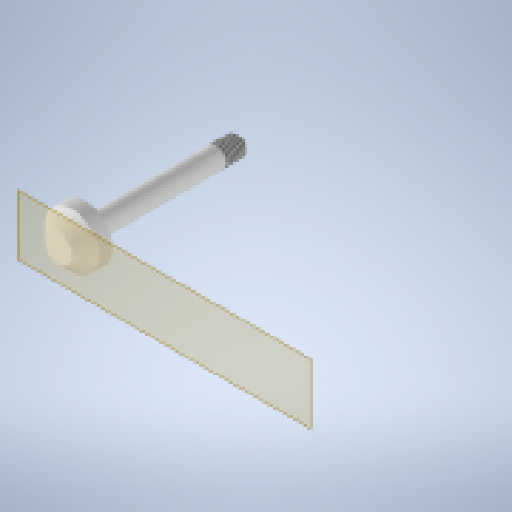
# Autodesk Inventor part: sornik1
Saved by Autodesk Inventor 2024 (Build 280153000, 153)
## iProperties
Created: 2023-10-02
Part Number: sornik1
Material: Generic
Document SubType Name: Modeling
Designer: jebes windows
Density: 1 g/cm^3
Appearance: Default
Author: jebes windows
Autodesk Inventor part; units mm, degrees
ref_plane "YZ Plane" through (0, 0, 0) normal (1, 0, 0) x (0, 1, 0)
ref_plane "XZ Plane" through (0, 0, 0) normal (0, 1, 0) x (-1, 0, 0)
ref_plane "XY Plane" through (0, 0, 0) normal (0, 0, 1) x (1, 0, 0)
ref_plane "Work Plane1" through (0, 0, 0) normal (0, 0, 1) x (1, 0, 0)
sketch "Sketch1" plane through (0, 0, 0) normal (0, 0, 1) x (1, 0, 0)
  arc A0 (-3.1429, -28.5256) -> (3.1429, -28.5256) centre (0, -30.9999) ccw projected
  arc A1 (2.5, -26.6698) -> (3.1429, -28.5256) centre (5.5, -26.6698) ccw projected
  line L0 (2.5, -4.3301) -> (2.5, -26.6698) projected
  arc A2 (3.1429, -2.4743) -> (2.5, -4.3301) centre (5.5, -4.3301) ccw projected
  arc A3 (3.1429, -2.4743) -> (-3.1429, -2.4743) centre (0, 0.0001) ccw projected
  arc A4 (-2.5, -4.3301) -> (-3.1429, -2.4743) centre (-5.5, -4.3301) ccw projected
  line L1 (-2.5, -4.3301) -> (-2.5, -26.6698) projected
  arc A5 (-3.1429, -28.5256) -> (-2.5, -26.6698) centre (-5.5, -26.6698) ccw projected
  circle A6 centre (0, -30.9999) radius 1.75 projected
  circle A7 centre (0, 0.0001) radius 1.75 projected
  circle A8 centre (0, 0.0001) radius 1.5
  point P0 (0, 0)
  dimension "d0" = 3
  constraints: 1 centre point, 1 coincident
  measures "d0" diameter of A8
extrude "Extrusion1" add sketch "Sketch1" against normal blind 27 contours A8
sketch "Sketch2" plane through (0, 0.0001, 0) normal (0, 0, 1) x (1, 0, 0)
  arc A0 (-3.1429, -28.5256) -> (3.1429, -28.5256) centre (0, -31) ccw projected
  arc A1 (2.5, -26.6699) -> (3.1429, -28.5256) centre (5.5, -26.6699) ccw projected
  line L0 (2.5, -4.3301) -> (2.5, -26.6699) projected
  arc A2 (3.1429, -2.4744) -> (2.5, -4.3301) centre (5.5, -4.3301) ccw projected
  arc A3 (3.1429, -2.4744) -> (-3.1429, -2.4744) centre (0, 0) ccw projected
  arc A4 (-2.5, -4.3301) -> (-3.1429, -2.4744) centre (-5.5, -4.3301) ccw projected
  line L1 (-2.5, -4.3301) -> (-2.5, -26.6699) projected
  arc A5 (-3.1429, -28.5256) -> (-2.5, -26.6699) centre (-5.5, -26.6699) ccw projected
  circle A6 centre (0, -31) radius 1.75 projected
  circle A7 centre (0, 0) radius 1.75 projected
  circle A8 centre (0, 0) radius 4
  point P0 (0, -0.0001)
  point P1 (4, 0)
  point P2 (3.1429, -2.4744)
  constraints: 1 centre point, 1 coincident, 1 concentric
extrude "Extrusion2" add sketch "Sketch2" against normal blind 4 contours A3 A8 | A7
chamfer "Chamfer1" distance 2 angle 45 1 edges at (-3.1429, 2.4744, 0)
thread "Thread1" size "M3x0.5" class "6g" standard "ISO Metric profile" length 4 offset 19
chamfer "Chamfer2" distance 1 angle 45 1 edges at (-1.5, 0.0001, -27)
body "Solid1"
